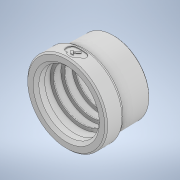
# Autodesk Inventor part: H32_R50_Zyclone
Saved by Autodesk Inventor 2020.2 (Build 242310000, 310)
## iProperties
Created: 2020-06-02
Part Number: H32_R50_Zyclone
Material: Generisch
Document SubType Name: Modeling
Designer: Rudi
Density: 1 g/cm^3
Appearance: Vorgabe
DN_Hose: 32,000 mm
d0: 32,000 mm
d2: 38,000 mm
d3: 42,000 mm
d4: 25,000 mm
Author: Rudi
Autodesk Inventor part; units mm, degrees
ref_plane "YZ Plane" through (0, 0, 0) normal (1, 0, 0) x (0, 1, 0)
ref_plane "XY Plane" through (0, 0, 0) normal (0, 0, 1) x (1, 0, 0)
sketch "Skizze1" plane through (0, 0, 0) normal (1, 0, 0) x (0, 1, 0)
  line L0 (16, 2) -> (19, 2)
  line L1 (19, 2) -> (21, 27)
  line L2 (21, 27) -> (25.5, 27)
  line L3 (16, 0) -> (16, 2)
  line L4 (0, 0) -> (0, 31.16)
  line L5 (25.5, 27) -> (24.9, 0)
  line L6 (24.9, 0) -> (16, 0)
  dimension "d0" = 32
  dimension "d2" = 38
  dimension "d3" = 42
  dimension "d4" = 25
  dimension "d7" = 49.8
  dimension "d8" = 51
  constraints: 14 end point, 2 horizontal, 1 coincident, 1 parallel, 1 vertical
  measures "d0" diameter of L3 L4
  measures "d2" diameter of L0.end L4
  measures "d3" diameter of L1.end L4
  measures "d4" distance between parallel lines of L0 L2
  measures "d7" diameter of L5.end L4
  measures "d8" diameter of L2.end L4
revolve "Umdrehung1" add sketch "Skizze1" angle 360 about axis through (0, 0, 0) along (0, 0, 1)
sketch "Skizze2" plane through (0, 0, 0) normal (1, 0, 0) x (0, 1, 0)
  line L0 (21, 33) -> (27.75, 33)
  line L1 (27.75, 33) -> (27.75, 21)
  line L2 (27.75, 21) -> (25.3357, 19.6061)
  line L3 (25.5, 27) -> (24.9, 0) projected
  line L4 (0, 0) -> (0, 41.2663)
  line L5 (21, 33) -> (21, 27)
  line L6 (19, 2) -> (21, 27) construction
  line L7 (-25.5, 27) -> (25.5, 27) projected
  dimension "d10" = 55.5
  dimension "d11" = 12
  dimension "d12" = 6
  dimension "d54" = 60
  constraints: 10 end point, 2 vertical, 1 perpendicular, 1 point on line
  measures "d10" diameter of L1 L4
  measures "d11" distance of L0.end L1.end
  measures "d12" distance between parallel lines of L0 L7
  measures "d54" angle of L2 L1
revolve "Umdrehung2" add sketch "Skizze2" angle 360 about axis through (0, 0, 0) along (0, 0, 1)
ref_plane "Arbeitsebene1" through (0, 37, 0) normal (0, 1, 0) x (-1, 0, 0)
sketch "Skizze3" plane through (0, 37, 0) normal (0, 1, 0) x (-1, 0, 0)
  arc A0 (4, 23) -> (3.489, 28.9562) centre (4, 26) ccw
  arc A1 (-3.9195, 27.7986) -> (-4, 23) centre (-4, 25.4) ccw
  line L0 (-33.0761, 23) -> (42.2204, 23) construction
  arc A2 (3.489, 28.9562) -> (-3.9195, 27.7986) centre (0, 27) ccw
  line L1 (0.1456, 27.5355) -> (1.1355, 26.5456)
  line L2 (1.1355, 26.5456) -> (-1.4101, 24)
  line L3 (-1.4101, 24) -> (-2.4, 24.9899)
  line L4 (-2.4, 24.9899) -> (0.1456, 27.5355)
  line L5 (-0.7029, 28.6669) -> (1.8426, 26.1213)
  line L6 (1.8426, 26.1213) -> (2.8326, 27.1113)
  line L7 (2.8326, 27.1113) -> (0.9941, 28.9497)
  line L8 (0.9941, 28.9497) -> (-0.7029, 28.6669)
  line L9 (-0.7029, 28.6669) -> (-0.6871, 28.6827) construction
  line L10 (-4, 23) -> (4, 23)
  line L11 (-13.9492, 33) -> (-13.9492, 21) construction
  line L12 (-27.75, 33) -> (27.75, 33) construction
  line L13 (-27.75, 21) -> (27.75, 21) construction
  point P0 (0, 0)
  point P1 (-4, 27.088)
  point P2 (-13.9492, 27)
  dimension "d15" = 4.8
  dimension "d16" = 6
  dimension "d17" = 4
  dimension "d18" = 4
  dimension "d19" = 4
  dimension "d20" = 4
  dimension "d21" = 45
  dimension "d22" = 1.4
  dimension "d23" = 3.6
  dimension "d24" = 2.6
  dimension "d25" = 1.4
  dimension "d26" = 0.8
  dimension "d27" = 1
  dimension "d28" = 0.2
  dimension "d29" = 1.6
  dimension "d30" = 1
  constraints: 25 end point, 6 point on circle, 4 perpendicular, 4 point on line, 3 centre point, 3 parallel, 2 tangent, 2 vertical alignment, 1 coincident, 1 horizontal, 1 horizontal alignment, 1 midpoint, 1 vertical
  measures "d15" diameter of A1
  measures "d16" diameter of A0
  measures "d17" horizontal distance of point (0, 27) A1.centre
  measures "d18" horizontal distance of A0.centre point (0, 27)
  measures "d19" distance from line of L0 point (0, 27)
  measures "d20" radius of A2
  measures "d21" angle of L0 L2
  measures "d22" distance of L2.end L3.end
  measures "d23" distance of L1.end L2.end
  measures "d24" distance of L6.end L7.end
  measures "d25" distance of L5.end L6.end
  measures "d26" distance from line of L5.end L2
  measures "d27" distance from line of L7.end L9
  measures "d28" distance between parallel lines of L5 L1
  measures "d29" horizontal distance of L3.end A1.centre
  measures "d30" distance from line of L2.end L0
emboss "Prägen1" sketch "Skizze3" operation cut depth 0.5 direction (0, 1, 0) wrap yes faces at (2.2329, 27.66, 25)
ref_plane "Arbeitsebene2" through (0, -42, 0) normal (0, -1, 0) x (1, 0, 0)
sketch "Skizze4" plane through (0, -42, 0) normal (0, -1, 0) x (1, 0, 0)
  line L0 (-9.2449, 28.8237) -> (9.2449, 28.8237) construction
  line L1 (9.2449, 28.8237) -> (9.2449, 25.1763) construction
  line L2 (9.2449, 25.1763) -> (-9.2449, 25.1763) construction
  line L3 (-9.2449, 25.1763) -> (-9.2449, 28.8237) construction
  line L4 (-21, 33) -> (21, 33) construction
  line L5 (-13.8816, 33) -> (-13.8816, 21) construction
  line L6 (-27.75, 21) -> (27.75, 21) construction
  line L7 (-14.5122, 23) -> (-15.5754, 23)
  line L8 (-15.5754, 23) -> (-15.5754, 26.9157)
  line L9 (-15.5754, 26.9157) -> (-19.2577, 26.9157)
  line L10 (-19.2577, 26.9157) -> (-19.2577, 23)
  line L11 (-19.2577, 23) -> (-20.3209, 23)
  line L12 (-20.3209, 23) -> (-20.3209, 31)
  line L13 (-20.3209, 31) -> (-19.2577, 31)
  line L14 (-19.2577, 31) -> (-19.2577, 27.8622)
  line L15 (-19.2577, 27.8622) -> (-15.5754, 27.8622)
  line L16 (-15.5754, 27.8622) -> (-15.5754, 31)
  line L17 (-15.5754, 31) -> (-14.5122, 31)
  line L18 (-14.5122, 31) -> (-14.5122, 23)
  spline S0 degree 2 poles (-10.9595, 30.2415) (-11.2512, 30.2415) (-11.8282, 30.0989) (-12.107, 29.9887) knots 0 0 0 1 2 2 2
  spline S1 degree 2 poles (-12.107, 29.9887) (-12.3663, 29.8784) (-12.7488, 29.6451) (-12.8979, 29.5413) knots 0 0 0 1 2 2 2
  line L19 (-12.8979, 29.5413) -> (-12.9627, 29.5413)
  line L20 (-12.9627, 29.5413) -> (-12.9627, 30.6759)
  spline S2 degree 2 poles (-12.9627, 30.6759) (-12.6126, 30.8639) (-11.4133, 31.1686) (-10.8752, 31.1686) knots 0 0 0 1 2 2 2
  spline S3 degree 2 poles (-10.8752, 31.1686) (-10.3306, 31.1686) (-9.5203, 30.9481) (-9.1896, 30.7147) knots 0 0 0 1 2 2 2
  spline S4 degree 2 poles (-9.1896, 30.7147) (-8.8395, 30.4619) (-8.4765, 29.7293) (-8.4765, 29.2366) knots 0 0 0 1 2 2 2
  spline S5 degree 2 poles (-8.4765, 29.2366) (-8.4765, 28.5754) (-9.3452, 27.577) (-9.9546, 27.4473) knots 0 0 0 1 2 2 2
  line L21 (-9.9546, 27.4473) -> (-9.9546, 27.3695)
  spline S6 degree 2 poles (-9.9546, 27.3695) (-9.7018, 27.3177) (-9.1248, 27.0843) (-8.8784, 26.8509) knots 0 0 0 1 2 2 2
  spline S7 degree 2 poles (-8.8784, 26.8509) (-8.6321, 26.624) (-8.3209, 25.8979) (-8.3209, 25.3728) knots 0 0 0 1 2 2 2
  spline S8 degree 2 poles (-8.3209, 25.3728) (-8.3209, 24.8347) (-8.6904, 23.9206) (-9.0276, 23.5705) knots 0 0 0 1 2 2 2
  spline S9 degree 2 poles (-9.0276, 23.5705) (-9.3776, 23.2075) (-10.3695, 22.8314) (-10.9984, 22.8314) knots 0 0 0 1 2 2 2
  spline S10 degree 2 poles (-10.9984, 22.8314) (-11.6013, 22.8314) (-12.7812, 23.1232) (-13.1831, 23.3241) knots 0 0 0 1 2 2 2
  line L22 (-13.1831, 23.3241) -> (-13.1831, 24.4587)
  line L23 (-13.1831, 24.4587) -> (-13.1053, 24.4587)
  spline S11 degree 2 poles (-13.1053, 24.4587) (-12.7682, 24.2123) (-11.6272, 23.7585) (-11.0632, 23.7585) knots 0 0 0 1 2 2 2
  spline S12 degree 2 poles (-11.0632, 23.7585) (-10.7326, 23.7585) (-10.0713, 23.966) (-9.8509, 24.2058) knots 0 0 0 1 2 2 2
  spline S13 degree 2 poles (-9.8509, 24.2058) (-9.637, 24.4457) (-9.41, 25.0162) (-9.41, 25.4506) knots 0 0 0 1 2 2 2
  spline S14 degree 2 poles (-9.41, 25.4506) (-9.41, 25.8849) (-9.6629, 26.4489) (-9.8898, 26.611) knots 0 0 0 1 2 2 2
  spline S15 degree 2 poles (-9.8898, 26.611) (-10.1167, 26.7731) (-10.7326, 26.8963) (-11.0956, 26.8963) knots 0 0 0 1 2 2 2
  line L24 (-11.0956, 26.8963) -> (-11.5494, 26.8963)
  line L25 (-11.5494, 26.8963) -> (-11.5494, 27.7844)
  line L26 (-11.5494, 27.7844) -> (-11.1929, 27.7844)
  spline S16 degree 2 poles (-11.1929, 27.7844) (-10.4733, 27.7844) (-9.5656, 28.4716) (-9.5656, 29.1264) knots 0 0 0 1 2 2 2
  spline S17 degree 2 poles (-9.5656, 29.1264) (-9.5656, 29.4311) (-9.799, 29.8655) (-9.987, 29.9951) knots 0 0 0 1 2 2 2
  spline S18 degree 2 poles (-9.987, 29.9951) (-10.188, 30.1313) (-10.6807, 30.2415) (-10.9595, 30.2415) knots 0 0 0 1 2 2 2
  line L27 (-2.1815, 23) -> (-7.1151, 23)
  line L28 (-7.1151, 23) -> (-7.1151, 24.1345)
  spline S19 degree 2 poles (-7.1151, 24.1345) (-6.5835, 24.6337) (-5.637, 25.5608) (-5.1831, 26.06) knots 0 0 0 1 2 2 2
  spline S20 degree 2 poles (-5.1831, 26.06) (-4.269, 27.0648) (-3.6013, 28.2707) (-3.6013, 28.9125) knots 0 0 0 1 2 2 2
  spline S21 degree 2 poles (-3.6013, 28.9125) (-3.6013, 29.2496) (-3.8088, 29.7553) (-3.9968, 29.9173) knots 0 0 0 1 2 2 2
  spline S22 degree 2 poles (-3.9968, 29.9173) (-4.1848, 30.0794) (-4.6775, 30.2415) (-4.9757, 30.2415) knots 0 0 0 1 2 2 2
  spline S23 degree 2 poles (-4.9757, 30.2415) (-5.2609, 30.2415) (-5.8444, 30.0989) (-6.1102, 29.9887) knots 0 0 0 1 2 2 2
  spline S24 degree 2 poles (-6.1102, 29.9887) (-6.3371, 29.8979) (-6.7585, 29.6386) (-6.8882, 29.5478) knots 0 0 0 1 2 2 2
  line L29 (-6.8882, 29.5478) -> (-6.9465, 29.5478)
  line L30 (-6.9465, 29.5478) -> (-6.9465, 30.6888)
  spline S25 degree 2 poles (-6.9465, 30.6888) (-6.6159, 30.8509) (-5.4295, 31.1686) (-4.8979, 31.1686) knots 0 0 0 1 2 2 2
  spline S26 degree 2 poles (-4.8979, 31.1686) (-3.7763, 31.1686) (-2.5122, 29.9822) (-2.5122, 28.9708) knots 0 0 0 1 2 2 2
  spline S27 degree 2 poles (-2.5122, 28.9708) (-2.5122, 28.4976) (-2.7326, 27.7066) (-2.9271, 27.3695) knots 0 0 0 1 2 2 2
  spline S28 degree 2 poles (-2.9271, 27.3695) (-3.1216, 27.0194) (-3.6856, 26.3323) (-3.9968, 26.0016) knots 0 0 0 1 2 2 2
  spline S29 degree 2 poles (-3.9968, 26.0016) (-4.5024, 25.4506) (-5.7407, 24.2707) (-6.1102, 23.9271) knots 0 0 0 1 2 2 2
  line L31 (-6.1102, 23.9271) -> (-2.1815, 23.9271)
  line L32 (-2.1815, 23.9271) -> (-2.1815, 23)
  line L33 (1.8185, 26.0146) -> (-1.2091, 26.0146)
  line L34 (-1.2091, 26.0146) -> (-1.2091, 26.987)
  line L35 (-1.2091, 26.987) -> (1.8185, 26.987)
  line L36 (1.8185, 26.987) -> (1.8185, 26.0146)
  line L37 (9.2998, 23) -> (7.919, 23)
  line L38 (7.919, 23) -> (5.3906, 26.1831)
  line L39 (5.3906, 26.1831) -> (4.1718, 26.1831)
  line L40 (4.1718, 26.1831) -> (4.1718, 23)
  line L41 (4.1718, 23) -> (3.1086, 23)
  line L42 (3.1086, 23) -> (3.1086, 31)
  line L43 (3.1086, 31) -> (5.1702, 31)
  spline S30 degree 2 poles (5.1702, 31) (5.8574, 31) (6.7844, 30.8509) (7.2058, 30.5786) knots 0 0 0 1 2 2 2
  spline S31 degree 2 poles (7.2058, 30.5786) (7.6272, 30.3063) (8.1135, 29.4571) (8.1135, 28.8282) knots 0 0 0 1 2 2 2
  spline S32 degree 2 poles (8.1135, 28.8282) (8.1135, 27.953) (7.2188, 26.7666) (6.4538, 26.4814) knots 0 0 0 1 2 2 2
  line L44 (6.4538, 26.4814) -> (9.2998, 23)
  spline S33 degree 2 poles (7.0049, 28.7439) (7.0049, 29.094) (6.7585, 29.6321) (6.4992, 29.8071) knots 0 0 0 1 2 2 2
  spline S34 degree 2 poles (6.4992, 29.8071) (6.2723, 29.9562) (5.6694, 30.0794) (5.2285, 30.0794) knots 0 0 0 1 2 2 2
  line L45 (5.2285, 30.0794) -> (4.1718, 30.0794)
  line L46 (4.1718, 30.0794) -> (4.1718, 27.0713)
  line L47 (4.1718, 27.0713) -> (5.1053, 27.0713)
  spline S35 degree 2 poles (5.1053, 27.0713) (5.5656, 27.0713) (6.2982, 27.2334) (6.5511, 27.4862) knots 0 0 0 1 2 2 2
  spline S36 degree 2 poles (6.5511, 27.4862) (6.7844, 27.7066) (7.0049, 28.329) (7.0049, 28.7439) knots 0 0 0 1 2 2 2
  spline S37 degree 2 poles (14.5575, 25.5413) (14.5575, 24.9643) (14.188, 23.9789) (13.8509, 23.6159) knots 0 0 0 1 2 2 2
  spline S38 degree 2 poles (13.8509, 23.6159) (13.5138, 23.2528) (12.5089, 22.8314) (11.8865, 22.8314) knots 0 0 0 1 2 2 2
  spline S39 degree 2 poles (11.8865, 22.8314) (11.316, 22.8314) (10.201, 23.0843) (9.7925, 23.2853) knots 0 0 0 1 2 2 2
  line L48 (9.7925, 23.2853) -> (9.7925, 24.4198)
  line L49 (9.7925, 24.4198) -> (9.8703, 24.4198)
  spline S40 degree 2 poles (9.8703, 24.4198) (9.9935, 24.329) (10.4538, 24.0956) (10.7326, 23.9919) knots 0 0 0 1 2 2 2
  spline S41 degree 2 poles (10.7326, 23.9919) (11.0502, 23.8817) (11.5754, 23.7585) (11.906, 23.7585) knots 0 0 0 1 2 2 2
  spline S42 degree 2 poles (11.906, 23.7585) (12.2301, 23.7585) (12.8395, 23.9919) (13.06, 24.2447) knots 0 0 0 1 2 2 2
  spline S43 degree 2 poles (13.06, 24.2447) (13.2609, 24.4846) (13.4684, 25.1199) (13.4684, 25.5478) knots 0 0 0 1 2 2 2
  spline S44 degree 2 poles (13.4684, 25.5478) (13.4684, 25.9757) (13.235, 26.5203) (13.0146, 26.7018) knots 0 0 0 1 2 2 2
  spline S45 degree 2 poles (13.0146, 26.7018) (12.7877, 26.9028) (12.1135, 27.0713) (11.705, 27.0713) knots 0 0 0 1 2 2 2
  spline S46 degree 2 poles (11.705, 27.0713) (11.2642, 27.0713) (10.389, 26.9352) (10.1232, 26.8768) knots 0 0 0 1 2 2 2
  line L50 (10.1232, 26.8768) -> (10.1232, 31)
  line L51 (10.1232, 31) -> (14.5122, 31)
  line L52 (14.5122, 31) -> (14.5122, 30.06)
  line L53 (14.5122, 30.06) -> (11.154, 30.06)
  line L54 (11.154, 30.06) -> (11.154, 27.9271)
  spline S47 degree 2 poles (11.154, 27.9271) (11.3485, 27.953) (11.7245, 27.9724) (11.8801, 27.9724) knots 0 0 0 1 2 2 2
  spline S48 degree 2 poles (11.8801, 27.9724) (12.4959, 27.9724) (13.3452, 27.7715) (13.7342, 27.4733) knots 0 0 0 1 2 2 2
  spline S49 degree 2 poles (13.7342, 27.4733) (14.1297, 27.175) (14.5575, 26.2674) (14.5575, 25.5413) knots 0 0 0 1 2 2 2
  spline S50 degree 2 poles (20.6904, 27) (20.6904, 24.8476) (19.4392, 22.8314) (18.1361, 22.8314) knots 0 0 0 1 2 2 2
  spline S51 degree 2 poles (18.1361, 22.8314) (16.8136, 22.8314) (15.5754, 24.8865) (15.5754, 26.9935) knots 0 0 0 1 2 2 2
  spline S52 degree 2 poles (15.5754, 26.9935) (15.5754, 29.1588) (16.8266, 31.1621) (18.1361, 31.1621) knots 0 0 0 1 2 2 2
  spline S53 degree 2 poles (18.1361, 31.1621) (19.4522, 31.1621) (20.6904, 29.0875) (20.6904, 27) knots 0 0 0 1 2 2 2
  spline S54 degree 2 poles (19.316, 24.5624) (19.4716, 24.9579) (19.6013, 26.1767) (19.6013, 27) knots 0 0 0 1 2 2 2
  spline S55 degree 2 poles (19.6013, 27) (19.6013, 27.8233) (19.4716, 29.0357) (19.3096, 29.4441) knots 0 0 0 1 2 2 2
  spline S56 degree 2 poles (19.3096, 29.4441) (19.1475, 29.8525) (18.5835, 30.2739) (18.1361, 30.2739) knots 0 0 0 1 2 2 2
  spline S57 degree 2 poles (18.1361, 30.2739) (17.6888, 30.2739) (17.1118, 29.8525) (16.9433, 29.4311) knots 0 0 0 1 2 2 2
  spline S58 degree 2 poles (16.9433, 29.4311) (16.7812, 29.0227) (16.6645, 27.778) (16.6645, 26.9935) knots 0 0 0 1 2 2 2
  spline S59 degree 2 poles (16.6645, 26.9935) (16.6645, 26.1507) (16.7682, 25.0227) (16.9368, 24.5818) knots 0 0 0 1 2 2 2
  spline S60 degree 2 poles (16.9368, 24.5818) (17.0924, 24.1669) (17.6694, 23.7196) (18.1361, 23.7196) knots 0 0 0 1 2 2 2
  spline S61 degree 2 poles (18.1361, 23.7196) (18.577, 23.7196) (19.154, 24.141) (19.316, 24.5624) knots 0 0 0 1 2 2 2
  point P0 (0, 0)
  point P1 (0, 28.8237)
  point P2 (-9.2449, 27)
  point P3 (-13.8816, 27)
  constraints: 3 midpoint, 2 end point, 2 point on line, 1 horizontal alignment, 1 vertical, 1 vertical alignment, 2 other
emboss "Prägen2" sketch "Skizze4" operation cut depth 0.5 direction (0, -1, 0) wrap yes faces at (10.7803, 25.5705, 26.5373) (0.4215, 27.7468, 26.3085) (-1.5576, 27.7063, 27.0655)
chamfer "Fase1" distance 1 angle 45 2 edges at (0, -27.75, 21) (0, -27.75, 33)
chamfer "Fase2" distance 2 angle 45 1 edges at (0, -21, 33)
sketch "Skizze5" plane through (0, 0, 0) normal (0, 1, 0) x (-1, 0, 0)
  line L0 (-19, 2) -> (-21, 27) projected
  line L1 (-21, 27) -> (-19.2205, 26.5168)
  line L2 (-20.8405, 25.0064) -> (-19.1605, 25.7663)
  arc A0 (-19.1605, 25.7663) -> (-19.2205, 26.5168) centre (-19.3254, 26.1308) ccw
  point P0 (0, 0)
  dimension "d43" = 2
  dimension "d44" = 2
  dimension "d45" = 0.4
  constraints: 4 end point, 2 point on circle, 2 tangent, 1 centre point, 1 equal length, 1 point on line
  measures "d43" distance of L0.end L2.start
  measures "d45" radius of A0
coil "Spirale1" sketch "Skizze5" operation add axis through (0, 0, -10) along (0, 0, -1) pitch 7 turns 3 hand left taper -4.57
chamfer "Fase3" distance 0.5 angle 45 3 edges at (0, -24.9, 0) (0, -16, 0) (0, -16, 2)
equation "\"d0\" = DN_Hose"
equation "\"d15\" = 1.2 * Scale"
equation "\"d16\" = 1.5 * Scale"
equation "\"d17\" = Scale"
equation "\"d18\" = Scale"
equation "\"d19\" = Scale"
equation "\"d20\" = Scale"
equation "\"d22\" = 0.35 * Scale"
equation "\"d23\" = 0.9 * Scale"
equation "\"d24\" = 0.65 * Scale"
equation "\"d25\" = 0.35 * Scale"
equation "\"d26\" = 0.2 * Scale"
equation "\"d27\" = 0.25 * Scale"
equation "\"d28\" = 0.05 * Scale"
equation "\"d29\" = 0.4 * Scale"
equation "\"d30\" = 0.25 * Scale"
equation "\"DN_Hose\" = 32"
equation "\"Scale\" = 4"
